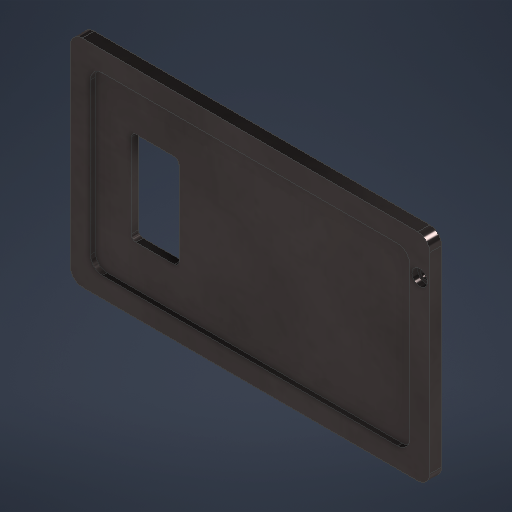
# Autodesk Inventor part: panel-suport
Saved by Autodesk Inventor 2026.2 (Build 302298010, 298A)
## iProperties
Created: 2026-04-07
Part Number: panel-suport
Material: Generic
Document SubType Name: Modeling
Designer: Aluno
Density: 1 g/cm^3
Appearance: Anodized - Subtle Dark Bronze
Author: Aluno
Autodesk Inventor part; units mm, degrees
ref_plane "YZ Plane" through (0, 0, 0) normal (1, 0, 0) x (0, 1, 0)
ref_plane "XZ Plane" through (0, 0, 0) normal (0, 1, 0) x (-1, 0, 0)
ref_plane "XY Plane" through (0, 0, 0) normal (0, 0, 1) x (1, 0, 0)
sketch "Sketch1" plane through (0, 0, 0) normal (0, 0, 1) x (1, 0, 0)
  line L0 (-75, 45) -> (75, 45)
  line L1 (75, 45) -> (75, -45)
  line L2 (75, -45) -> (-75, -45)
  line L3 (-75, -45) -> (-75, 45)
  line L4 (-75, 45) -> (75, -45) construction
  line L5 (75, 45) -> (-75, -45) construction
  point P0 (0, 0)
  dimension "d0" = 150
  dimension "d1" = 90
  constraints: 12 end point, 2 midpoint, 2 parallel, 1 horizontal, 1 perpendicular
  measures "d0" distance of L1.end L2.end
  measures "d1" distance of L0.end L1.end
extrude "Extrusion1" add sketch "Sketch1" along normal blind 5
fillet "Fillet1" radius 5 4 edges at (75, 45, 2.5) (75, -45, 2.5) (-75, -45, 2.5) (-75, 45, 2.5)
sketch "Sketch2" plane through (0, 0, 5) normal (0, 0, 1) x (1, 0, 0)
  line L0 (-61.6, -36.6) -> (61.6, -36.6)
  line L1 (66.6, -31.6) -> (66.6, 31.6)
  line L2 (61.6, 36.6) -> (-61.6, 36.6)
  line L3 (-66.6, 31.6) -> (-66.6, -31.6)
  line L4 (-66.6, -36.6) -> (66.6, 36.6) construction
  line L5 (66.6, -36.6) -> (-66.6, 36.6) construction
  arc A0 (-61.6, 36.6) -> (-66.6, 31.6) centre (-61.6, 31.6) ccw
  arc A1 (-66.6, -31.6) -> (-61.6, -36.6) centre (-61.6, -31.6) ccw
  arc A2 (61.6, -36.6) -> (66.6, -31.6) centre (61.6, -31.6) ccw
  arc A3 (66.6, 31.6) -> (61.6, 36.6) centre (61.6, 31.6) ccw
  point P0 (0, 0)
  dimension "d5" = 133.2
  dimension "d6" = 73.2
  dimension "d9" = 5
  constraints: 12 end point, 8 point on circle, 8 point on line, 8 tangent, 4 centre point, 3 equal radius, 2 midpoint, 2 parallel, 1 horizontal, 1 perpendicular
  measures "d5" distance of L5.end L4.end
  measures "d6" distance of L5.start L4.end
  measures "d9" radius of A0
extrude "Extrusion2" cut sketch "Sketch2" against normal blind 2
sketch "Sketch3" plane through (0, 0, 5) normal (0, 0, 1) x (1, 0, 0)
  line L0 (66.6, 31.6) -> (66.6, -31.6) projected
  line L1 (66.6, 0) -> (75, 0) construction
  line L2 (75, -40) -> (75, 40) projected
  line L3 (70.8, 0) -> (70.8, 28.8336) construction
  circle A0 centre (70.8, 28.8336) radius 3.25
  point P0 (0, 0)
  dimension "d10" = 6.5
  constraints: 4 end point, 3 midpoint, 1 centre point, 1 coincident, 1 vertical
  measures "d10" diameter of A0
extrude "Extrusion3" cut sketch "Sketch3" against normal blind 2.4
sketch "Sketch4" plane through (70.8, 28.8336, 2.6) normal (0, 0, 1) x (1, 0, 0)
  circle A0 centre (0, 0) radius 2
  point P0 (-70.8, -28.8336)
  dimension "d13" = 4
  constraints: 1 centre point
  measures "d13" diameter of A0
extrude "Extrusion4" cut sketch "Sketch4" against normal blind 15
sketch "Sketch7" plane through (0, 0, 3) normal (0, 0, 1) x (1, 0, 0)
  line L0 (-66.6, -31.6) -> (-66.6, 31.6) projected
  line L1 (-66.6, 0.4) -> (-51.6, 0.4) construction
  line L2 (61.6, -36.6) -> (-61.6, -36.6) projected
  line L3 (-51.6, -36.6) -> (-51.6, -19.6) construction
  line L4 (-51.6, -36.6) -> (-34.6, -36.6) construction
  line L5 (-66.6, 19.9067) -> (-31.6, 19.9067) construction
  line L6 (-31.6, -17.6) -> (-31.6, 19.4) construction
  line L7 (-31.6, -36.6) -> (5.4, -36.6) construction
  line L8 (-49.6, -19.6) -> (-33.6, -19.6)
  line L9 (-31.6, -19.6) -> (-31.6, 17.4)
  line L10 (-33.6, 19.4) -> (-49.6, 19.4)
  line L11 (-51.6, 17.4) -> (-51.6, -17.6)
  arc A0 (-49.6, 19.4) -> (-51.6, 17.4) centre (-49.6, 17.4) ccw
  arc A1 (-31.6, 17.4) -> (-33.6, 19.4) centre (-33.6, 17.4) ccw
  arc A2 (-33.6, -19.6) -> (-31.6, -17.6) centre (-33.6, -17.6) ccw
  arc A3 (-51.6, -17.6) -> (-49.6, -19.6) centre (-49.6, -17.6) ccw
  point P0 (0, 0)
  point P1 (-67, -23.834)
  point P2 (-31.6, -17.6)
  dimension "d30" = 17
  dimension "d31" = 90
  dimension "d34" = 56
  dimension "d35" = 90
  dimension "d36" = 15
  dimension "d37" = 35
  dimension "d38" = 2
  constraints: 20 end point, 8 point on circle, 8 point on line, 8 tangent, 5 horizontal, 4 centre point, 4 perpendicular, 3 equal radius, 2 parallel, 1 vertical, 3 other
  measures "d30" distance of L3.start L3.end
  measures "d31" angle of L4 L3
  measures "d34" distance of L7.start L6.end
  measures "d35" angle of L7 L6
  measures "d38" radius of A0
extrude "Extrusion6" cut sketch "Sketch7" against normal blind 8.25
body "Solid1"
